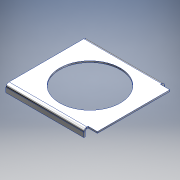
# Autodesk Inventor part: Turret Base Plate
Saved by Autodesk Inventor 2019.4 (Build 234330000, 330)
## iProperties
Created: 2020-01-11
Part Number: Turret Base Plate
Material: Aluminum 6061
Document SubType Name: Sheet Metal
Designer: admin
Density: 2.7 g/cm^3
Sheet Metal Rule: Default_mm
Appearance: Aluminum - Flat
Author: admin
Autodesk Inventor part; units mm, degrees
ref_plane "YZ Plane" through (0, 0, 0) normal (1, 0, 0) x (0, 1, 0)
ref_plane "XZ Plane" through (0, 0, 0) normal (0, 1, 0) x (-1, 0, 0)
ref_plane "XY Plane" through (0, 0, 0) normal (0, 0, 1) x (1, 0, 0)
sketch "Sketch1" plane through (0, 0, 0) normal (0, 1, 0) x (-1, 0, 0)
  circle A0 centre (0, 0) radius 97.5
  line L0 (-140, 130) -> (140, 130)
  line L1 (140, 130) -> (140, -130)
  line L2 (140, -130) -> (-140, -130)
  line L3 (-140, -130) -> (-140, 130)
  line L4 (-140, 130) -> (140, -130) construction
  line L5 (140, 130) -> (-140, -130) construction
  dimension "d0" = 195
  dimension "d1" = 280
  dimension "d2" = 260
  measures "d0" diameter of A0
  measures "d1" distance of L1.end L2.end
  measures "d2" distance of L0.end L1.end
extrude "Plate1" add sketch "Sketch1" along normal blind 5
sketch "Sketch2" plane through (-140, 5, 125) normal (0, 0, 1) x (1, 0, 0)
  line L0 (280, 0) -> (0, 0)
  line L1 (0, 0) -> (0, -25)
  line L2 (0, -25) -> (280, -25)
  line L3 (280, -25) -> (280, 0)
  constraints: 6 end point, 1 horizontal, 1 perpendicular, 1 vertical
edge flange "Flange1" height 25 angle 90 thickness 5 bend radius 5 thickness toward (0, 0, 1) relief straight relief width 5 relief depth 2.5 corner gap 5 corner form 0 edges at (0, 0, 130) (0, 0, -130) wall of the first edge with corners at (140, 5, 125) (-140, 5, 125) (-140, -20, 125) (140, -20, 125)
bend "Bend1"
corner "Corner1"
unfold all bends "Unfold1" k factor 0.44 fixed face at (-125.8333, 5, 0)
sketch "Sketch3" plane through (0, 5, 0) normal (0, 1, 0) x (1, 0, 0)
  line L0 (140, -146.3097) -> (-140, -146.3097) projected
  line L1 (110, -146.3097) -> (110, -116.3097)
  line L2 (110, -116.3097) -> (140, -116.3097)
  line L3 (140, 120) -> (140, -120) projected
  line L4 (140, -120) -> (140, -131.3097) projected
  line L5 (140, -131.3097) -> (140, -146.3097) projected
  line L6 (-140, 146.3097) -> (140, 146.3097) projected
  line L7 (140, 146.3097) -> (110, 146.3097)
  line L8 (110, 146.3097) -> (110, 116.3097)
  line L9 (110, 116.3097) -> (140, 116.3097)
  line L10 (140, 116.3097) -> (140, 146.3097)
  point P0 (0, 0)
  dimension "d14" = 30
  dimension "d15" = 30
  dimension "d16" = 30
  dimension "d17" = 30
  constraints: 12 end point, 2 parallel, 2 perpendicular, 2 point on line, 1 horizontal, 1 vertical
  measures "d14" distance of L1.end L2.end
  measures "d15" distance of L1.start L1.end
  measures "d16" distance of L9.end L8.end
  measures "d17" distance of L8.end L7.end
extrude "Extrusion1" cut sketch "Sketch3" against normal through all
refold all bends "Refold1"
equation "\"d3\" = Thickness"
equation "\"d4\" = BendReliefWidth"
equation "\"d5\" = BendReliefDepth"
equation "\"d6\" = MinimumRemnant"
equation "\"d7\" = TransitionRadius"
equation "\"d10\" = BendRadius"
equation "\"d11\" = CornerReliefSize"
equation "\"d12\" = GapSize"
equation "\"d13\" = JacobiRadiusSize"
equation "\"BendRadius\" = Thickness"
equation "\"BendReliefWidth\" = Thickness"
equation "\"BendReliefDepth\" = 0.5 * Thickness"
equation "\"TransitionRadius\" = BendRadius"
equation "\"JacobiRadiusSize\" = BendRadius"
equation "\"GapSize\" = Thickness"
equation "\"Thickness\" = 5"
equation "\"MinimumRemnant\" = 10"
equation "\"CornerReliefSize\" = 20"
body "Solid1"
